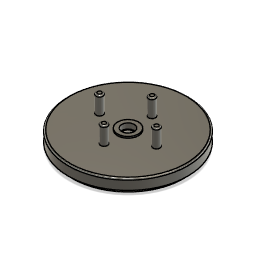
Magnet glueing jig v6 (Autodesk Fusion 360 design; units mm, degrees)
Autodesk Fusion 360 part; units mm, degrees
sketch "Sketch1" plane through (0, 0, 0) normal (0, 1, 0) x (1, 0, 0)
  line L0 (-9.55, 0) -> (9.55, 0) construction
  line L1 (0, 8.05) -> (0, -8.05) construction
  circle A0 centre (0, 8.05) radius 1.15
  circle A1 centre (0, -8.05) radius 1.15
  circle A2 centre (-9.55, 0) radius 1.15
  circle A3 centre (9.55, 0) radius 1.15
  circle A4 centre (0, 0) radius 13.75 construction
  circle A5 centre (0, 0) radius 20
  circle A6 centre (0, 0) radius 2.1
  circle A7 centre (0, 0) radius 1.25
  circle A8 centre (0, 8.05) radius 1.25 construction
  circle A9 centre (9.55, 0) radius 1.25 construction
  circle A10 centre (-9.55, 0) radius 1.25 construction
  circle A11 centre (0, -8.05) radius 1.25 construction
  circle A12 centre (0, 0) radius 3.5
  point P0 (-8.3, 0)
  point P1 (0, 6.8)
  point P2 (8.3, 0)
  point P3 (0, -6.8)
  dimension "d3" = 2.3
  dimension "d4" = 2.3
  dimension "d5" = 2.3
  dimension "d6" = 2.3
  dimension "d7" = 27.5
  dimension "d8" = 40
  dimension "d9" = 4.2
  dimension "d10" = 2.5
  dimension "d24" = 2.5
  dimension "d25" = 2.5
  dimension "d26" = 2.5
  dimension "d27" = 2.5
  dimension "d28" = 13.6
  dimension "d29" = 16.6
  dimension "d30" = 19.1
  dimension "d31" = 7
  constraint horizontal L0
  constraint midpoint L0 A4.centre
  constraint coincident A4.centre A5.centre
  constraint perpendicular L0 L1
  constraint coincident A4.centre L1
  constraint midpoint L1 A4.centre
  constraint coincident L1.start A0.centre
  constraint coincident L1.end A1.centre
  constraint coincident L0.start A2.centre
  constraint coincident L0.end A3.centre
  constraint concentric A4 A6
  constraint concentric A0 A8
  constraint concentric A3 A9
  constraint concentric A2 A10
  constraint concentric A1 A11
  constraint coincident A10 P0
  constraint coincident L0 P0
  constraint coincident A8 P1
  constraint coincident L1 P1
  constraint coincident A9 P2
  constraint coincident L0 P2
  constraint coincident A11 P3
  constraint coincident L1 P3
  constraint concentric A4 A12
  measures "d3" diameter of A0
  measures "d4" diameter of A1
  measures "d5" diameter of A2
  measures "d6" diameter of A3
  measures "d7" diameter of A4
  measures "d8" diameter of A5
  measures "d9" diameter of A6
  measures "d10" diameter of A7
  measures "d24" diameter of A8
  measures "d25" diameter of A9
  measures "d26" diameter of A10
  measures "d27" diameter of A11
  measures "d28" distance of P1 P3
  measures "d29" distance of P0 P2
  measures "d30" distance of L0.end L0.start
  measures "d31" diameter of A12
extrude "Extrude1" add sketch "Sketch1" along normal blind 5 contours A5 | A12
extrude "Extrude2" add sketch "Sketch1" along normal blind 3.7 contours A6
extrude "Extrude3" add sketch "Sketch1" along normal blind 11 contours A0 | A1 | A2 | A3
fillet "Fillet1" radius 0.5 4 edges at (-1.0722, 11, -7.6341) (8.4778, 11, 0.4159) (-1.0722, 11, 8.4659) (-10.6222, 11, 0.4159)
fillet "Fillet2" radius 0.5 1 edges at (-1.1654, 3.7, -0.452)
fillet "Fillet3" radius 0.5 1 edges at (-18.6465, 5, 7.2323)
chamfer "Chamfer1" distance 1.5 angle 45 2 edges at (-18.6465, 0, 7.2323) (-1.1654, 0, -0.452)
extrude "Extrude4" add sketch "Sketch1" along normal blind 5.5 contours A12
